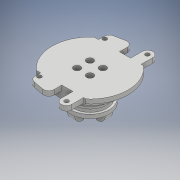
# Autodesk Inventor part: ax12_base
Saved by Autodesk Inventor 2017 (Build 210142000, 142)
## iProperties
Created: 2016-03-16
Part Number: ax12_base
Material: Generic
Document SubType Name: Modeling
Designer: alist
Density: 1 g/cm^3
Appearance: Default
Author: alist
Autodesk Inventor part; units mm, degrees
ref_plane "YZ Plane" through (0, 0, 0) normal (1, 0, 0) x (0, 1, 0)
ref_plane "XZ Plane" through (0, 0, 0) normal (0, 1, 0) x (-1, 0, 0)
ref_plane "XY Plane" through (0, 0, 0) normal (0, 0, 1) x (1, 0, 0)
sketch "Sketch1" plane through (0, 0, 0) normal (0, 0, 1) x (1, 0, 0)
  line L0 (35.4703, 11) -> (41.4703, 11) construction
  line L1 (35.4703, -71) -> (41.4703, -71) construction
  line L2 (39.6026, 0) -> (39.6026, -30) construction
  circle A0 centre (19.9026, -30) radius 11
  line L3 (63.6359, -30) -> (-19.5974, -30) construction
  line L4 (39.6026, -30) -> (39.6026, -60) construction
  line L5 (39.6026, 0) -> (45.5979, 0)
  line L6 (-5.7927, 0) -> (39.6026, 0)
  line L7 (-5.7927, -60) -> (39.6026, -60)
  line L8 (39.6026, -60) -> (45.5979, -60)
  line L9 (49.4646, -60) -> (45.5979, -60) construction
  line L10 (49.4646, -60) -> (45.5979, -60) construction
  line L11 (45.5979, 0) -> (45.5979, -60) construction
  line L12 (-5.7927, 0) -> (-5.7927, -60) construction
  arc A1 (-5.7927, 0) -> (-5.7927, -60) centre (19.9026, -30) ccw
  arc A2 (45.5979, -60) -> (45.5979, 0) centre (19.9026, -30) ccw
  dimension "d0" = 22
  dimension "d1" = 19.7
  dimension "d102" = 39.5
  dimension "d103" = 39.5
  constraints: 18 end point, 5 horizontal, 5 point on circle, 3 centre point, 2 coincident, 2 perpendicular, 2 point on line, 2 vertical, 1 collinear
  measures "d0" diameter of A0
  measures "d1" distance from line of L2 A0.centre
  measures "d102" radius of A2
  measures "d103" radius of A1
extrude "Extrusion1" add sketch "Sketch1" along normal blind 5 contours A0 | L5 A2 L8 L7 A1 L6
sketch "Sketch2" plane through (0, 0, 0) normal (0, 0, -1) x (-1, 0, 0)
  line L0 (-45.5979, 0) -> (5.7927, 0) projected
  arc A0 (-45.5979, 0) -> (-45.5979, -60) centre (-19.9026, -30) ccw projected
  line L1 (5.7927, -60) -> (-45.5979, -60) projected
  arc A1 (5.7927, -60) -> (5.7927, 0) centre (-19.9026, -30) ccw projected
  line L2 (-41.4703, -71) -> (-35.4703, -71) construction
  line L3 (-41.4703, 11) -> (-35.4703, 11) construction
  line L4 (-38.4703, -71) -> (-38.4703, 11) construction
  line L5 (-59.4026, -30) -> (19.5974, -30) construction
  circle A2 centre (-19.9026, -30) radius 26.5
  point P0 (0, 0)
  dimension "d6" = 53
  constraints: 4 end point, 2 midpoint, 2 point on circle, 1 centre point, 1 coincident, 1 horizontal
  measures "d6" diameter of A2
extrude "Extrusion2" add sketch "Sketch2" along normal blind 8
chamfer "Chamfer1" distance 1 angle 45 1 edges at (46.4026, -30, -8)
chamfer "Chamfer2" distance 10 distance2 8.5 1 edges at (59.4026, -30, -8) measured on face at (58.9026, -30, -8)
sketch "Sketch3" plane through (0, 0, 5) normal (0, 0, 1) x (1, 0, 0)
  circle A0 centre (1.2406, -64) radius 2.15 projected
  line L0 (20.5421, -60) -> (-1.4421, -60)
  circle A1 centre (37.6089, -72.0643) radius 2.15 projected
  line L1 (43.1313, -60) -> (32.1313, -60)
  line L2 (43.1313, -72.1598) -> (43.1313, -60)
  line L3 (32.1313, -60) -> (32.1313, -72.1598)
  arc A2 (32.1313, -72.1598) -> (43.1313, -72.1598) centre (37.6313, -72.1598) ccw
  arc A3 (14.0389, -73.3768) -> (20.5421, -67.9691) centre (15.0421, -67.9691) ccw
  line L4 (20.5421, -67.9691) -> (20.5421, -60)
  line L5 (-1.4421, -60) -> (-1.4421, -65.9313)
  arc A4 (-1.4421, -65.9313) -> (3.0546, -71.339) centre (4.0579, -65.9313) ccw
  line L6 (3.0546, -71.339) -> (14.0389, -73.3768)
  point P0 (0, 0)
  constraints: 14 end point, 6 point on circle, 3 centre point
extrude "Extrusion3" add sketch "Sketch3" against normal blind 5
ref_plane "Work Plane1" through (-5.7927, -30, 5) normal (0, 1, 0) x (1, 0, 0)
mirror "Mirror1" about plane through (-5.7927, -30, 5) normal (0, 1, 0) of "Extrusion3"
sketch "Sketch4" plane through (19.9026, -30, 0) normal (0, 0, -1) x (-1, 0, 0)
  circle A0 centre (0, 0) radius 26.5 projected
  circle A1 centre (0, 0) radius 26.5 projected
  circle A2 centre (0, 0) radius 22.5
  point P0 (19.9026, 30)
  dimension "d22" = 4
  constraints: 1 centre point
  measures "d22" radial gap between concentric circles of A0 A2
extrude "Extrusion4" add sketch "Sketch4" along normal blind 1.75 draft -45 contours A2
sketch "Sketch5" plane through (19.9026, -30, -1.75) normal (0, 0, -1) x (-1, 0, 0)
  circle A0 centre (0, 0) radius 20.75 projected
  circle A1 centre (0, 0) radius 17.5
  point P0 (19.9026, 30)
  dimension "d25" = 35
  constraints: 1 centre point, 1 coincident
  measures "d25" diameter of A1
extrude "Extrusion5" add sketch "Sketch5" along normal blind 6.9 contours A1
sketch "Sketch6" plane through (19.9026, -30, -8.65) normal (0, 0, -1) x (-1, 0, 0)
  circle A0 centre (0, 0) radius 17.5 projected
  circle A1 centre (0, 0) radius 9.5 construction
  circle A2 centre (6.7175, -6.7175) radius 2.15
  line L0 (23.5934, 0) -> (-20.2582, 0) construction
  line L1 (0, 0) -> (10.2597, -10.2597) construction
  line L2 (0, 0) -> (14.5094, 0) construction
  circle A3 centre (6.7175, 6.7175) radius 2.15
  circle A4 centre (-6.7175, 6.7175) radius 2.15
  circle A5 centre (-6.7175, -6.7175) radius 2.15
  point P0 (19.9026, 30)
  dimension "d28" = 8
  dimension "d29" = 4.3
  dimension "d30" = 45
  dimension "d33" = 360
  constraints: 6 end point, 4 centre point, 2 horizontal, 2 point on line, 1 equal length, 12 other
  measures "d29" diameter of A2
  measures "d30" angle of L1 L2
extrude "Extrusion6" cut sketch "Sketch6" against normal through all contours A2 | A3 | A4 | A5
sketch "Sketch7" plane through (0, 0, 5) normal (0, 0, 1) x (1, 0, 0)
  circle A0 centre (13.1851, -36.7175) radius 2.15 projected
  circle A1 centre (13.1851, -23.2825) radius 2.15 projected
  circle A2 centre (26.6201, -23.2825) radius 2.15 projected
  circle A3 centre (26.6201, -36.7175) radius 2.15 projected
  circle A4 centre (13.1851, -36.7175) radius 3.5
  circle A5 centre (13.1851, -23.2825) radius 3.5
  circle A6 centre (26.6201, -23.2825) radius 2.15 projected
  circle A7 centre (26.6201, -23.2825) radius 3.5
  circle A8 centre (26.6201, -36.7175) radius 3.5
  point P0 (0, 0)
  dimension "d38" = 7
  dimension "d39" = 7
  dimension "d40" = 7
  dimension "d41" = 7
  constraints: 4 centre point, 4 coincident
  measures "d38" diameter of A4
  measures "d39" diameter of A5
  measures "d40" diameter of A7
  measures "d41" diameter of A8
extrude "Extrusion7" cut sketch "Sketch7" against normal blind 5.35 contours A0 | A1 | A2 | A3 | A4 | A5 | A7 | A8
chamfer "Chamfer4" distance 1.35 angle 45 4 edges at (23.1201, -36.7175, -0.35) (9.6851, -36.7175, -0.35) (9.6851, -23.2825, -0.35) (23.1201, -23.2825, -0.35)
sketch "Sketch8" plane through (19.9026, -30, -8.65) normal (0, 0, -1) x (-1, 0, 0)
  circle A0 centre (-6.7175, -6.7175) radius 2.15 projected
  circle A1 centre (6.7175, 6.7175) radius 2.15 projected
  circle A2 centre (6.7175, -6.7175) radius 2.15 projected
  circle A3 centre (-6.7175, 6.7175) radius 2.15 projected
  circle A4 centre (0, 0) radius 20
  point P0 (19.9026, 30)
  dimension "d47" = 40
  constraints: 5 centre point
  measures "d47" diameter of A4
extrude "Extrusion8" add sketch "Sketch8" along normal blind 7 separate body
sketch "Sketch9" plane through (19.9026, -30, -15.65) normal (0, 0, -1) x (-1, 0, 0)
  circle A0 centre (0, 0) radius 17.5 projected
  circle A1 centre (-6.7175, 6.7175) radius 2.15 projected
  circle A2 centre (6.7175, -6.7175) radius 2.15 projected
  circle A3 centre (6.7175, 6.7175) radius 2.15 projected
  circle A4 centre (-6.7175, -6.7175) radius 2.15 projected
  point P0 (19.9026, 30)
  constraints: 4 centre point
extrude "Extrusion9" add sketch "Sketch9" along normal blind 3.9 separate body
sketch "Sketch10" plane through (19.9026, -30, -19.55) normal (0, 0, -1) x (-1, 0, 0)
  circle A0 centre (-6.7175, -6.7175) radius 2.15 projected
  circle A1 centre (6.7175, 6.7175) radius 2.15 projected
  circle A2 centre (6.7175, -6.7175) radius 2.15 projected
  circle A3 centre (-6.7175, 6.7175) radius 2.15 projected
  circle A4 centre (0, 0) radius 17.5
  point P0 (19.9026, 30)
  dimension "d52" = 35
  constraints: 5 centre point
  measures "d52" diameter of A4
extrude "Extrusion10" add sketch "Sketch10" along normal blind 3 separate body
sketch "Sketch11" plane through (19.9026, -30, -22.55) normal (0, 0, -1) x (-1, 0, 0)
  circle A0 centre (-6.7175, 6.7175) radius 2.15 projected
  circle A1 centre (6.7175, -6.7175) radius 2.15 projected
  circle A2 centre (6.7175, 6.7175) radius 2.15 projected
  circle A3 centre (-6.7175, -6.7175) radius 2.15 projected
  circle A4 centre (0, 0) radius 20
  point P0 (19.9026, 30)
  constraints: 5 centre point
extrude "Extrusion11" add sketch "Sketch11" along normal blind 4 bodies 4
sketch "Sketch12" plane through (19.9026, -30, -26.55) normal (0, 0, -1) x (-1, 0, 0)
  arc A0 (15.5919, 3.7781) -> (15.5919, -3.7781) centre (0, 0) ccw
  circle A1 centre (6.7175, -6.7175) radius 2.15 construction
  line L0 (5.6416, -2.7022) -> (9.6569, -3.7781)
  line L1 (9.6569, -3.7781) -> (10.7328, -7.7934)
  line L2 (10.7328, -7.7934) -> (9.2631, -9.2631)
  line L3 (7.7934, -10.7328) -> (3.7781, -9.6569)
  line L4 (3.7781, -9.6569) -> (2.7022, -5.6416)
  line L5 (2.7022, -5.6416) -> (5.6416, -2.7022)
  line L6 (19.6901, -2.9983) -> (2.1604, -20.528) construction
  line L7 (11.3442, -11.3442) -> (0, 0) construction
  line L8 (9.2631, -9.2631) -> (7.7934, -10.7328)
  line L9 (0, 0) -> (13.7633, 0) construction
  line L10 (9.6569, 3.7781) -> (5.6416, 2.7022)
  line L11 (5.6416, 2.7022) -> (2.7022, 5.6416)
  line L12 (2.7022, 5.6416) -> (3.7781, 9.6569)
  line L13 (3.7781, 9.6569) -> (7.7934, 10.7328)
  line L14 (7.7934, 10.7328) -> (9.2631, 9.2631)
  line L15 (10.7328, 7.7934) -> (9.6569, 3.7781)
  line L16 (9.2631, 9.2631) -> (10.7328, 7.7934)
  line L17 (-3.7781, 9.6569) -> (-2.7022, 5.6416)
  line L18 (-2.7022, 5.6416) -> (-5.6416, 2.7022)
  line L19 (-5.6416, 2.7022) -> (-9.6569, 3.7781)
  line L20 (-9.6569, 3.7781) -> (-10.7328, 7.7934)
  line L21 (-10.7328, 7.7934) -> (-9.2631, 9.2631)
  line L22 (-7.7934, 10.7328) -> (-3.7781, 9.6569)
  line L23 (-9.2631, 9.2631) -> (-7.7934, 10.7328)
  line L24 (-9.6569, -3.7781) -> (-5.6416, -2.7022)
  line L25 (-5.6416, -2.7022) -> (-2.7022, -5.6416)
  line L26 (-2.7022, -5.6416) -> (-3.7781, -9.6569)
  line L27 (-3.7781, -9.6569) -> (-7.7934, -10.7328)
  line L28 (-7.7934, -10.7328) -> (-9.2631, -9.2631)
  line L29 (-10.7328, -7.7934) -> (-9.6569, -3.7781)
  line L30 (-9.2631, -9.2631) -> (-10.7328, -7.7934)
  arc A2 (19.6399, -3.7781) -> (19.6399, 3.7781) centre (0, 0) ccw
  line L31 (0, -16.0431) -> (0, 16.0431)
  line L32 (16.0431, 0) -> (-16.0431, 0)
  line L33 (19.6399, -3.7781) -> (9.6569, -3.7781)
  line L34 (19.6399, 3.7781) -> (9.6569, 3.7781)
  line L35 (-19.6399, -3.7781) -> (-9.6569, -3.7781)
  line L36 (-19.6399, 3.7781) -> (-9.6569, 3.7781)
  line L37 (3.7781, -19.6399) -> (3.7781, -9.6569)
  line L38 (-3.7781, -19.6399) -> (-3.7781, -9.6569)
  line L39 (3.7781, 19.6399) -> (3.7781, 9.6569)
  line L40 (-3.7781, 19.6399) -> (-3.7781, 9.6569)
  arc A3 (2.8997, -19.7887) -> (3.7781, -19.6399) centre (0, 0) ccw
  arc A4 (-3.7781, -19.6399) -> (2.8997, -19.7887) centre (0, 0) ccw
  arc A5 (-19.6399, 3.7781) -> (-19.6399, -3.7781) centre (0, 0) ccw
  arc A6 (3.7781, 19.6399) -> (-3.7781, 19.6399) centre (0, 0) ccw
  arc A7 (19.6399, 3.7781) -> (19.5842, 4.057) centre (0, 0) ccw
  point P0 (19.9026, 30)
  point P1 (-15.5919, -3.7781)
  point P2 (-15.5919, 3.7781)
  point P3 (3.7781, -15.5919)
  point P4 (-3.7781, -15.5919)
  point P5 (3.7781, 15.5919)
  point P6 (-3.7781, 15.5919)
  dimension "d57" = 7.2
  dimension "d59" = 45
  dimension "d62" = 360
  constraints: 82 end point, 28 point on circle, 14 point on line, 7 centre point, 7 symmetric about line, 2 coincident, 2 horizontal, 2 vertical, 1 collinear, 1 perpendicular, 1 tangent, 71 other
  measures "d57" distance between parallel lines of L4 L1
  measures "d59" angle of L7 L9
extrude "Extrusion12" cut sketch "Sketch12" against normal blind 4 contours L10 L11 L12 L13 L14 L16 L15 | L17 L18 L19 L20 L21 L23 L22 | L1 L2 L8 L3 L4 L5 L0 | L27 L28 L30 L29 L24 L25 L26 bodies 4
extrude "Extrusion13" add sketch "Sketch12" along normal blind 8 contours L34 A2 L33 L0 L5 L4 L37 A0 L31 L39 L12 L11 L10 | A0 L40 A6 L39 | L31 L32 A0 L36 L19 L18 L17 L40 | L31 A0 L38 L26 L25 L24 L35 L32 | A0 L35 A5 L36 | A0 L37 A3 A4 L38 bodies 4
sketch "Sketch13" plane through (19.9026, -30, -34.55) normal (0, 0, -1) x (-1, 0, 0)
  circle A0 centre (0, 0) radius 8 construction
  circle A1 centre (8, 0) radius 1.15
  circle A2 centre (0, 8) radius 1.15
  circle A3 centre (-8, 0) radius 1.15
  circle A4 centre (0, -8) radius 1.15
  point P0 (19.9026, 30)
  dimension "d69" = 16
  dimension "d70" = 2.3
  dimension "d73" = 360
  constraints: 4 centre point, 1 horizontal alignment, 11 other
  measures "d70" diameter of A1
extrude "Extrusion14" cut sketch "Sketch13" against normal up to next bodies 4
sketch "Sketch14" plane through (19.9026, -30, -19.55) normal (0, 0, 1) x (1, 0, 0)
  circle A0 centre (8, 0) radius 1.15 construction
  circle A1 centre (0, -8) radius 1.15 construction
  circle A2 centre (-8, 0) radius 1.15 construction
  circle A3 centre (0, 8) radius 1.15 construction
  circle A4 centre (8, 0) radius 2
  circle A5 centre (0, 8) radius 2
  circle A6 centre (-8, 0) radius 2
  circle A7 centre (0, -8) radius 2
  point P0 (-19.9026, 30)
  point P1 (0, 0)
  dimension "d77" = 4
  dimension "d80" = 360
  constraints: 4 centre point, 1 coincident, 9 other
  measures "d77" diameter of A4
extrude "Extrusion15" cut sketch "Sketch14" against normal up to surface (7 mm away) bodies 4
sketch "Sketch15" plane through (19.9026, -30, -34.55) normal (0, 0, -1) x (-1, 0, 0)
  circle A0 centre (0, 0) radius 11.1
  point P0 (19.9026, 30)
  dimension "d84" = 22.2
  constraints: 1 centre point
  measures "d84" diameter of A0
extrude "Extrusion16" cut sketch "Sketch15" against normal blind 1 bodies 4
hole "Hole1" at (19.9026, -30, -33.55) direction (0, 0, 1) diameter 5 end through all counterbore diameter 10 counterbore depth 1 bodies 4
combine bodies "Combine1" operation type add bodies to combine 3 2
fillet "Fillet1" radius 8 4 edges at (39.9026, -30, -34.55) (19.9026, -10, -34.55) (-0.0974, -30, -34.55) (19.9026, -50, -34.55)
chamfer "Chamfer5" distance 1 angle 45 12 edges at (25.6884, -19.8052, -26.55) (29.1657, -20.7369, -26.55) (30.0975, -24.2142, -26.55) (14.1169, -19.8052, -26.55) (10.6395, -20.7369, -26.55) (9.7078, -24.2142, -26.55) (9.7078, -35.7858, -26.55) (10.6395, -39.2631, -26.55) (14.1169, -40.1948, -26.55) (30.0975, -35.7858, -26.55) (29.1657, -39.2631, -26.55) (25.6884, -40.1948, -26.55)
ref_plane "Work Plane2" through (-5.7927, -30, 5) normal (0, 1, 0) x (1, 0, 0)
